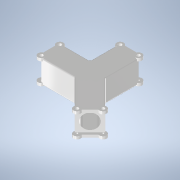
# Autodesk Inventor part: BracketV3
Saved by Autodesk Inventor 2022 (Build 260153000, 153)
## iProperties
Created: 2022-02-09
Part Number: BracketV3
Material: Generic
Document SubType Name: Modeling
Designer: ultra
Density: 1 g/cm^3
Appearance: Smooth - White
Author: ultra
Autodesk Inventor part; units mm, degrees
ref_plane "YZ Plane" through (0, 0, 0) normal (1, 0, 0) x (0, 1, 0)
ref_plane "XZ Plane" through (0, 0, 0) normal (0, 1, 0) x (-1, 0, 0)
ref_plane "XY Plane" through (0, 0, 0) normal (0, 0, 1) x (1, 0, 0)
sketch "Sketch1" plane through (0, 0, 0) normal (1, 0, 0) x (0, 1, 0)
  line L0 (0, 0) -> (41.5544, 0)
  line L1 (41.5544, 0) -> (41.5544, 37.0078)
  line L2 (41.5544, 37.0078) -> (0, 37.0078)
  line L3 (0, 37.0078) -> (0, 0)
  circle A0 centre (20.7772, 18.5039) radius 12.8778
  dimension "d0" = 41.5544
  dimension "d1" = 37.0078
  dimension "d2" = 25.7556
  constraints: 8 end point, 2 parallel, 1 centre point, 1 horizontal, 1 perpendicular
  measures "d0" distance of L2.end L1.end
  measures "d1" distance of L1.end L0.end
  measures "d2" diameter of A0
extrude "Extrusion1" add sketch "Sketch1" along normal blind 50.8
sketch "Sketch2" plane through (0, 0, 0) normal (0, 0, -1) x (-1, 0, 0)
  line L0 (-50.8, 0) -> (-50.8, 41.5544) projected
  line L1 (-50.8, 41.5544) -> (-87.8078, 41.5544)
  line L2 (-87.8078, 41.5544) -> (-87.8078, 0)
  line L3 (-87.8078, 0) -> (-50.8, 0)
  line L4 (-50.8, 0) -> (-50.8, 41.5544)
  circle A0 centre (-69.3039, 20.7772) radius 12.8778
  dimension "d5" = 37.0078
  dimension "d6" = 25.7556
  constraints: 8 end point, 2 parallel, 1 centre point, 1 horizontal, 1 perpendicular
  measures "d5" distance of L3.end L2.end
  measures "d6" diameter of A0
extrude "Extrusion2" add sketch "Sketch2" against normal up to surface (37.0078 mm away) contours L3 L2 L1 L0 | A0
sketch "Sketch3" plane through (0, 0, 0) normal (0, 0, -1) x (-1, 0, 0)
  line L0 (0, 41.5544) -> (-87.8078, 41.5544) projected
  line L1 (-87.8078, 41.5544) -> (-87.8078, 0) projected
  line L2 (0, 0) -> (-87.8078, 0) projected
  line L3 (0, 0) -> (-87.8078, 0) projected
  line L4 (-87.8078, 41.5544) -> (-50.8, 41.5544)
  line L5 (-50.8, 41.5544) -> (-50.8, 0)
  line L6 (-50.8, 0) -> (-87.8078, 0)
  line L7 (-87.8078, 0) -> (-87.8078, 41.5544)
  circle A0 centre (-69.3039, 20.7772) radius 12.8778
  point P0 (-50.8, 0)
  dimension "d9" = 37.0078
  dimension "d10" = 25.7556
  constraints: 8 end point, 2 parallel, 1 centre point, 1 horizontal, 1 perpendicular, 1 point on line
  measures "d9" distance of L5.end L6.end
  measures "d10" diameter of A0
extrude "Extrusion3" add sketch "Sketch3" along normal blind 50.8
sketch "Sketch4" plane through (0, 41.5544, 37.0078) normal (0, 1, 0) x (1, 0, 0)
  line L0 (0, 0) -> (87.8078, 0) projected
  line L1 (87.8078, 87.8078) -> (87.8078, 0) projected
  line L2 (50.8, 37.0078) -> (50.8, 87.8078) projected
  line L3 (87.8078, 0) -> (87.8078, 87.8078) projected
  line L4 (50.8, 37.0078) -> (87.8078, 0)
  line L5 (87.8078, 0) -> (123.1594, -36.4815)
  line L6 (87.8078, 0) -> (100.892, 13.0842)
  line L7 (0, 0) -> (87.8078, 0) projected
  line L8 (87.8078, 0) -> (74.7236, -13.0842)
  line L9 (100.892, 13.0842) -> (87.8078, 26.1685)
  line L10 (74.7236, -13.0842) -> (61.6393, 0)
  line L11 (100.892, 13.0842) -> (136.8086, -22.8323)
  line L12 (136.8086, -22.8323) -> (123.1594, -36.4815)
  line L13 (123.1594, -36.4815) -> (110.6401, -49.0008)
  line L14 (123.1594, -36.4815) -> (140.8643, -36.4815) construction
  line L15 (110.6401, -49.0008) -> (74.7236, -13.0842)
  dimension "d13" = 50.8
  dimension "d14" = 18.5039
  dimension "d15" = 18.5039
  dimension "d16" = 135
  constraints: 22 end point, 4 point on line, 3 perpendicular, 1 equal length, 1 horizontal
  measures "d13" distance of L0.end L5.end
  measures "d14" distance of L0.end L6.end
  measures "d15" distance of L0.end L8.end
  measures "d16" angle of L13 L14
extrude "Extrusion4" add sketch "Sketch4" against normal up to surface (41.5544 mm away)
sketch "Sketch5" plane through (136.8086, 0, 59.8401) normal (0.7071068, 0, 0.7071068) x (0.7071068, 0, -0.7071068)
  line L0 (-18.5039, 41.5544) -> (-18.5039, 0) projected
  circle A0 centre (-18.5039, 20.7772) radius 12.8778
  point P0 (-54.4249, 0)
  dimension "d19" = 25.7556
  constraints: 1 centre point, 1 midpoint
  measures "d19" diameter of A0
extrude "Extrusion5" cut sketch "Sketch5" against normal blind 76.2
sketch "Sketch6" plane through (0, 41.5544, 37.0078) normal (0, 1, 0) x (1, 0, 0)
  line L0 (0, 37.0078) -> (0, 0) projected
  line L1 (0, 0) -> (61.6393, 0) projected
  line L2 (61.6393, 0) -> (110.6401, -49.0008) projected
  line L3 (110.6401, -49.0008) -> (136.8086, -22.8323) projected
  line L4 (136.8086, -22.8323) -> (87.8078, 26.1685) projected
  line L5 (87.8078, 87.8078) -> (87.8078, 26.1685) projected
  line L6 (50.8, 87.8078) -> (87.8078, 87.8078) projected
  line L7 (50.8, 37.0078) -> (50.8, 87.8078) projected
  line L8 (0, 37.0078) -> (50.8, 37.0078) projected
  line L9 (0, 18.5039) -> (69.3039, 18.5039)
  line L10 (69.3039, 18.5039) -> (69.3039, 87.8078)
  line L11 (56.4261, 87.8078) -> (82.1817, 87.8078) projected
  line L12 (69.3039, 18.5039) -> (123.7244, -35.9166)
  circle A0 centre (2.4892, 2.879) radius 1.5875
  circle A1 centre (2.4892, 34.1288) radius 1.5875
  circle A2 centre (84.9288, 85.3186) radius 1.5875
  circle A3 centre (53.679, 85.3186) radius 1.5875
  circle A4 centre (110.9158, -45.2049) radius 1.5875
  circle A5 centre (133.0127, -23.108) radius 1.5875
  dimension "d22" = 3.175
  dimension "d23" = 3.175
  dimension "d24" = 2.4892
  dimension "d25" = 2.4892
  dimension "d26" = 2.879
  dimension "d27" = 2.879
  dimension "d28" = 3.175
  dimension "d29" = 3.175
  dimension "d30" = 2.4892
  dimension "d31" = 2.4892
  dimension "d32" = 2.879
  dimension "d33" = 2.879
  dimension "d34" = 3.175
  dimension "d35" = 3.175
  dimension "d36" = 2.4892
  dimension "d37" = 2.4892
  dimension "d38" = 2.879
  dimension "d39" = 2.879
  constraints: 6 centre point, 6 end point, 3 midpoint, 1 perpendicular
  measures "d22" diameter of A0
  measures "d23" diameter of A1
  measures "d24" distance from line of L0 A0.centre
  measures "d25" distance from line of L0 A1.centre
  measures "d26" distance from line of L1 A0.centre
  measures "d27" distance from line of L8 A1.centre
  measures "d28" diameter of A2
  measures "d29" diameter of A3
  measures "d30" vertical distance of L11.start A3.centre
  measures "d31" distance from line of L6 A2.centre
  measures "d32" distance from line of L5 A2.centre
  measures "d33" distance from line of L7 A3.centre
  measures "d34" diameter of A4
  measures "d35" diameter of A5
  measures "d36" distance from line of L3 A4.centre
  measures "d37" distance from line of L3 A5.centre
  measures "d38" distance from line of L4 A5.centre
  measures "d39" distance from line of L2 A4.centre
extrude "Extrusion6" cut sketch "Sketch6" against normal blind 50.8 contours A0 | A1 | A2 | A3 | A4 | A5
sketch "Sketch7" plane through (0, 41.5544, 37.0078) normal (0, 1, 0) x (1, 0, 0)
  circle A0 centre (2.4892, 2.879) radius 1.5875 projected
  circle A1 centre (110.9158, -45.2049) radius 1.5875 projected
  circle A2 centre (53.679, 85.3186) radius 1.5875 projected
  circle A3 centre (2.4892, 34.1288) radius 1.5875 projected
  circle A4 centre (84.9288, 85.3186) radius 1.5875 projected
  line L0 (0, 37.0078) -> (0, 0) projected
  line L1 (0, 0) -> (61.6393, 0) projected
  line L2 (61.6393, 0) -> (110.6401, -49.0008) projected
  line L3 (110.6401, -49.0008) -> (136.8086, -22.8323) projected
  line L4 (136.8086, -22.8323) -> (87.8078, 26.1685) projected
  line L5 (87.8078, 87.8078) -> (87.8078, 26.1685) projected
  line L6 (50.8, 87.8078) -> (87.8078, 87.8078) projected
  line L7 (50.8, 37.0078) -> (50.8, 87.8078) projected
  line L8 (0, 37.0078) -> (50.8, 37.0078) projected
  circle A5 centre (133.0127, -23.108) radius 1.5875 projected
  circle A6 centre (133.0127, -23.108) radius 6
  circle A7 centre (110.9158, -45.2049) radius 6
  circle A8 centre (2.4892, 2.879) radius 6
  circle A9 centre (2.4892, 34.1288) radius 6
  circle A10 centre (53.679, 85.3186) radius 6
  circle A11 centre (84.9288, 85.3186) radius 6
  point P0 (0, 8.3383)
  point P1 (7.7534, 0)
  point P2 (7.7534, 37.0078)
  point P3 (0, 28.6695)
  point P4 (59.1383, 87.8078)
  point P5 (50.8, 80.0544)
  point P6 (79.4695, 87.8078)
  point P7 (87.8078, 80.0544)
  point P8 (130.9126, -28.7284)
  point P9 (131.3262, -17.3499)
  point P10 (105.1577, -43.5184)
  point P11 (116.5362, -43.1048)
  dimension "d42" = 12
  dimension "d43" = 12
  dimension "d44" = 12
  dimension "d45" = 12
  dimension "d46" = 12
  dimension "d47" = 12
  constraints: 6 centre point, 6 coincident
  measures "d42" diameter of A6
  measures "d43" diameter of A7
  measures "d44" diameter of A8
  measures "d45" diameter of A9
  measures "d46" diameter of A10
  measures "d47" diameter of A11
extrude "Extrusion7" add sketch "Sketch7" against normal blind 4.7752 contours L0 A9 L8 | L0 L1 A8 | A10 L6 L7 | L2 L3 A7 | A11 L5 L6 | L3 L4 A6 picked at (-0.4033, 31.694) picked at (-0.4033, 5.3138) picked at (56.1138, 88.2111) picked at (106.9061, -45.8277) picked at (82.5067, 88.2271) picked at (133.3453, -26.876)
sketch "Sketch8" plane through (0, 0, 0) normal (0, -1, 0) x (1, 0, 0)
  circle A0 centre (2.4892, 34.1288) radius 1.5875 projected
  circle A1 centre (53.679, -48.3108) radius 1.5875 projected
  circle A2 centre (2.4892, 2.879) radius 1.5875 projected
  circle A3 centre (84.9288, -48.3108) radius 1.5875 projected
  line L0 (0, 37.0078) -> (0, 0) projected
  line L1 (0, 0) -> (50.8, 0) projected
  line L2 (50.8, 0) -> (50.8, -50.8) projected
  line L3 (87.8078, -50.8) -> (50.8, -50.8) projected
  line L4 (87.8078, 10.8393) -> (87.8078, -50.8) projected
  line L5 (136.8086, 59.8401) -> (87.8078, 10.8393) projected
  line L6 (110.6401, 86.0086) -> (136.8086, 59.8401) projected
  line L7 (61.6393, 37.0078) -> (110.6401, 86.0086) projected
  line L8 (0, 37.0078) -> (61.6393, 37.0078) projected
  circle A4 centre (110.9158, 82.2127) radius 1.5875 projected
  circle A5 centre (110.9158, 82.2127) radius 6
  circle A6 centre (133.0127, 60.1158) radius 1.5875 projected
  circle A7 centre (133.0127, 60.1158) radius 6
  circle A8 centre (84.9288, -48.3108) radius 6
  circle A9 centre (53.679, -48.3108) radius 6
  circle A10 centre (2.4892, 2.879) radius 6
  circle A11 centre (2.4892, 34.1288) radius 6
  point P0 (0, 8.3383)
  point P1 (7.7534, 0)
  point P2 (7.7534, 37.0078)
  point P3 (0, 28.6695)
  point P4 (116.5362, 80.1126)
  point P5 (105.1577, 80.5262)
  point P6 (131.3262, 54.3577)
  point P7 (130.9126, 65.7362)
  point P8 (87.8078, -43.0466)
  point P9 (79.4695, -50.8)
  point P10 (50.8, -43.0466)
  point P11 (59.1383, -50.8)
  dimension "d50" = 12
  constraints: 6 centre point, 6 coincident
  measures "d50" diameter of A5
extrude "Extrusion8" add sketch "Sketch8" against normal blind 4.7752 contours L0 A11 L8 | L0 L1 A10 | A5 L6 L7 | L2 L3 A9 | A7 L5 L6 | L3 L4 A8 picked at (-0.4033, 31.694) picked at (-0.4033, 5.3138) picked at (106.9061, 82.8355) picked at (56.1138, -51.2033) picked at (133.3453, 63.8838) picked at (82.5067, -51.2193)
sketch "Sketch9" plane through (0, 41.5544, 28.6695) normal (0, 1, 0) x (1, 0, 0)
  circle A0 centre (2.4892, -5.4593) radius 1.5875 projected
  circle A1 centre (110.9158, -53.5432) radius 1.5875 projected
  circle A2 centre (53.679, 76.9803) radius 1.5875 projected
  circle A3 centre (2.4892, 25.7905) radius 1.5875 projected
  circle A4 centre (133.0127, -31.4463) radius 1.5875 projected
  circle A5 centre (84.9288, 76.9803) radius 1.5875 projected
  arc A6 (0, 0) -> (7.7534, -8.3383) centre (2.4892, -5.4593) ccw projected
  arc A7 (105.1577, -51.8567) -> (116.5362, -51.443) centre (110.9158, -53.5432) ccw projected
  arc A8 (87.8078, 71.7161) -> (79.4695, 79.4695) centre (84.9288, 76.9803) ccw projected
  arc A9 (7.7534, 28.6695) -> (0, 20.3312) centre (2.4892, 25.7905) ccw projected
  circle A10 centre (110.9158, -53.5432) radius 2.925
  circle A11 centre (133.0127, -31.4463) radius 1.5875 projected
  circle A12 centre (133.0127, -31.4463) radius 2.925
  circle A13 centre (84.9288, 76.9803) radius 2.925
  circle A14 centre (53.679, 76.9803) radius 1.5875 projected
  circle A15 centre (53.679, 76.9803) radius 2.925
  circle A16 centre (2.4892, 25.7905) radius 2.925
  circle A17 centre (2.4892, -5.4593) radius 2.925
  point P0 (0, 28.6695)
  dimension "d53" = 5.85
  dimension "d54" = 5.85
  dimension "d55" = 5.85
  dimension "d56" = 5.85
  dimension "d57" = 5.85
  dimension "d58" = 5.85
  constraints: 6 centre point, 6 coincident
  measures "d53" diameter of A10
  measures "d54" diameter of A12
  measures "d55" diameter of A13
  measures "d56" diameter of A15
  measures "d57" diameter of A16
  measures "d58" diameter of A17
sketch "Sketch10" plane through (0, 0, -50.8) normal (0, 0, -1) x (-1, 0, 0)
  line L0 (-59.1383, 4.7752) -> (-50.8, 4.7752) projected
  line L1 (-50.8, 4.7752) -> (-50.8, 36.7792) projected
  line L2 (-50.8, 36.7792) -> (-59.1383, 36.7792) projected
  line L3 (-79.4695, 36.7792) -> (-87.8078, 36.7792) projected
  line L4 (-87.8078, 36.7792) -> (-87.8078, 4.7752) projected
  line L5 (-87.8078, 4.7752) -> (-79.4695, 4.7752) projected
  circle A0 centre (-69.3039, 20.7772) radius 12.8778 projected
  line L6 (-87.8078, 4.7752) -> (-50.8, 4.7752)
  line L7 (-50.8, 4.7752) -> (-50.8, 36.7792)
  line L8 (-50.8, 36.7792) -> (-87.8078, 36.7792)
  line L9 (-87.8078, 36.7792) -> (-87.8078, 4.7752)
  line L10 (-87.8078, 4.7752) -> (-50.8, 36.7792) construction
  line L11 (-50.8, 4.7752) -> (-87.8078, 36.7792) construction
  point P0 (0, 0)
  constraints: 12 end point, 2 midpoint, 2 parallel, 1 horizontal, 1 perpendicular
extrude "Extrusion9" cut sketch "Sketch10" against normal blind 5.0038
sketch "Sketch11" plane through (0, 0, 0) normal (-1, 0, 0) x (0, 0, 1)
  line L0 (28.6695, 4.7752) -> (37.0078, 4.7752) projected
  line L1 (37.0078, 36.7792) -> (37.0078, 4.7752) projected
  line L2 (37.0078, 36.7792) -> (28.6695, 36.7792) projected
  line L3 (8.3383, 36.7792) -> (0, 36.7792) projected
  line L4 (0, 4.7752) -> (0, 36.7792) projected
  line L5 (0, 4.7752) -> (8.3383, 4.7752) projected
  circle A0 centre (18.5039, 20.7772) radius 12.8778 projected
  line L6 (0, 4.7752) -> (37.0078, 4.7752)
  line L7 (37.0078, 4.7752) -> (37.0078, 36.7792)
  line L8 (37.0078, 36.7792) -> (0, 36.7792)
  line L9 (0, 36.7792) -> (0, 4.7752)
  line L10 (0, 4.7752) -> (37.0078, 36.7792) construction
  line L11 (37.0078, 4.7752) -> (0, 36.7792) construction
  point P0 (0, 0)
  constraints: 12 end point, 2 midpoint, 2 parallel, 1 horizontal, 1 perpendicular
extrude "Extrusion10" cut sketch "Sketch11" against normal blind 5.0038
sketch "Sketch12" plane through (130.9126, 36.7792, 65.7362) normal (0.7071068, 0, 0.7071068) x (0.7071068, 0, -0.7071068)
  line L0 (0, -32.004) -> (8.3383, -32.004) projected
  line L1 (8.3383, 0) -> (8.3383, -32.004) projected
  line L2 (8.3383, 0) -> (0, 0) projected
  line L3 (-20.3312, 0) -> (-28.6695, 0) projected
  line L4 (-28.6695, 0) -> (-28.6695, -32.004) projected
  line L5 (-28.6695, -32.004) -> (-20.3312, -32.004) projected
  circle A0 centre (-10.1656, -16.002) radius 12.8778 projected
  line L6 (-28.6695, -32.004) -> (8.3383, -32.004)
  line L7 (8.3383, -32.004) -> (8.3383, 0)
  line L8 (8.3383, 0) -> (-28.6695, 0)
  line L9 (-28.6695, 0) -> (-28.6695, -32.004)
  line L10 (-28.6695, -32.004) -> (8.3383, 0) construction
  line L11 (8.3383, -32.004) -> (-28.6695, 0) construction
  point P0 (-46.0866, -36.7792)
  point P1 (-20.3312, 0)
  point P2 (-20.3312, -32.004)
  constraints: 12 end point, 2 midpoint, 2 parallel, 1 horizontal, 1 perpendicular
extrude "Extrusion11" cut sketch "Sketch12" against normal blind 5.0038
extrude "Extrusion12" cut sketch "Sketch9" against normal blind 5.08
fillet "Fillet1" radius 3.175 15 edges at (50.8, 20.7772, 0) (29.2767, 41.5544, 0) (50.8, 41.5544, -21.5233) (50.8, 0, -21.5233) (29.2767, 0, 0) (34.6963, 41.5544, 37.0078) (83.3985, 41.5544, 58.767) (83.3985, 0, 58.767) (109.567, 41.5544, 32.5985) (109.567, 0, 32.5985) (87.8078, 41.5544, -16.1037) (87.8078, 0, -16.1037) (34.6963, 0, 37.0078) (61.6393, 20.7772, 37.0078) (87.8078, 20.7772, 10.8393)
sketch "Sketch13" plane through (0, 41.5544, 28.6695) normal (0, 1, 0) x (1, 0, 0)
  line L0 (59.1383, 79.4695) -> (79.4695, 79.4695) projected
  line L1 (0, 20.3312) -> (0, 0) projected
  line L2 (116.5362, -51.443) -> (130.9126, -37.0667) projected
  line L3 (78.9488, 18.7326) -> (60.7369, 0.5207) projected
  line L4 (79.4695, 79.4695) -> (59.1383, 79.4695) projected
  line L5 (69.3039, 79.4695) -> (69.3039, 9.0877)
  line L6 (69.3039, 9.0877) -> (123.1854, -44.7938)
  line L7 (130.9126, -37.0667) -> (116.5362, -51.443) projected
  line L8 (0, 10.1656) -> (69.3039, 10.1656)
  circle A0 centre (15.875, 10.1656) radius 6.35
  circle A1 centre (69.3039, 63.5945) radius 6.35
  circle A2 centre (111.9601, -33.5685) radius 6.35
  circle A3 centre (41.275, 10.1656) radius 6.35
  circle A4 centre (69.3039, 38.1945) radius 6.35
  circle A5 centre (93.9996, -15.608) radius 6.35
  circle A6 centre (76.0391, 2.3525) radius 6.35
  point P0 (0, 28.6695)
  dimension "d68" = 12.7
  dimension "d69" = 15.875
  dimension "d72" = 12.7
  dimension "d73" = 15.875
  dimension "d77" = 12.7
  dimension "d78" = 15.875
  dimension "d83" = 25.4
  dimension "d90" = 25.4
  dimension "d97" = 25.4
  constraints: 7 centre point, 6 end point, 6 point on line, 2 midpoint, 2 vertical, 1 horizontal, 1 perpendicular, 9 other
  measures "d68" diameter of A0
  measures "d69" distance from line of L1 A0.centre
  measures "d72" diameter of A1
  measures "d73" distance from line of L0 A1.centre
  measures "d77" diameter of A2
  measures "d78" distance from line of L2 A2.centre
  measures "d83" distance of A0.centre A3.centre
  measures "d90" distance of A1.centre A4.centre
  measures "d97" distance of A2.centre A5.centre
extrude "Extrusion13" [suppressed]
sketch "Sketch15" plane through (0, 0, 8.3383) normal (0, -1, 0) x (1, 0, 0)
  line L0 (79.4695, -59.1383) -> (59.1383, -59.1383) projected
  line L1 (0, 0) -> (0, 20.3312) projected
  line L2 (0, 11.0475) -> (68.3935, 11.0475)
  line L3 (68.3935, 11.0475) -> (68.3935, -59.1383)
  line L4 (68.3935, 11.0475) -> (138.5793, 11.0475) construction
  line L5 (65.9805, 6.2215) -> (70.8065, 6.2215)
  line L6 (70.8065, 6.2215) -> (70.8065, 15.8735)
  line L7 (70.8065, 15.8735) -> (65.9805, 15.8735)
  line L8 (65.9805, 15.8735) -> (65.9805, 6.2215)
  line L9 (65.9805, 6.2215) -> (70.8065, 15.8735) construction
  line L10 (70.8065, 6.2215) -> (65.9805, 15.8735) construction
  line L11 (62.8055, 3.0465) -> (73.9815, 3.0465)
  line L12 (73.9815, 3.0465) -> (73.9815, 19.0485)
  line L13 (73.9815, 19.0485) -> (62.8055, 19.0485)
  line L14 (62.8055, 19.0485) -> (62.8055, 3.0465)
  line L15 (62.8055, 3.0465) -> (73.9815, 19.0485) construction
  line L16 (73.9815, 3.0465) -> (62.8055, 19.0485) construction
  point P0 (0, -8.3383)
  dimension "d104" = 90
  dimension "d105" = 4.826
  dimension "d106" = 9.652
  dimension "d107" = 11.176
  dimension "d108" = 16.002
  constraints: 30 end point, 4 horizontal, 4 midpoint, 4 parallel, 3 perpendicular, 2 point on line
  measures "d104" angle of L3 L4
  measures "d105" distance of L7.end L6.end
  measures "d106" distance of L6.end L5.end
  measures "d107" distance of L13.end L12.end
  measures "d108" distance of L12.end L11.end
extrude "Extrusion14" add sketch "Sketch15" along normal blind 12.7 contours L14 L13 L12 L11 L3 L5 L6 L7 L8 L2 | L2 L8 L5 L3 L11 L14
sketch "Sketch16" plane through (73.9815, 0, 27.3868) normal (1, 0, 0) x (0, 0, -1)
  line L0 (0, 0) -> (0, -12.7) projected
  line L1 (16.002, -12.7) -> (0, -12.7) projected
  circle A0 centre (8.001, -7.112) radius 3.175
  point P0 (27.3868, 0)
  dimension "d111" = 6.35
  dimension "d112" = 8.001
  dimension "d113" = 5.588
  constraints: 1 centre point
  measures "d111" diameter of A0
  measures "d112" distance from line of L0 A0.centre
  measures "d113" distance from line of A0.centre L1
extrude "Extrusion15" cut sketch "Sketch16" against normal blind 279.4
equation "\"d7\" = d6"
body "Solid1"
